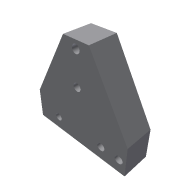
# Autodesk Inventor part: cellSTORM_chip_Adapter_screws
Saved by Autodesk Inventor 2019 (Build 230136000, 136)
## iProperties
Created: 2020-02-12
Part Number: cellSTORM_chip_Adapter_screws
Material: Generic
Document SubType Name: Modeling
Designer: diederichbenedict
Density: 1 g/cm^3
Appearance: Default
Author: diederichbenedict
Autodesk Inventor part; units mm, degrees
ref_plane "YZ Plane" through (0, 0, 0) normal (1, 0, 0) x (0, 1, 0)
ref_plane "XZ Plane" through (0, 0, 0) normal (0, 1, 0) x (-1, 0, 0)
ref_plane "XY Plane" through (0, 0, 0) normal (0, 0, 1) x (1, 0, 0)
sketch "Sketch1" plane through (0, 0, 0) normal (0, 0, 1) x (1, 0, 0)
  line L0 (18.5, -17.5) -> (-18.5, -17.5)
  line L1 (-18.5, -17.5) -> (-18.5, 17.5)
  line L2 (-18.5, 17.5) -> (18.5, 17.5)
  line L3 (18.5, 17.5) -> (18.5, -17.5)
  line L4 (18.5, -17.5) -> (-18.5, 17.5) construction
  line L5 (-18.5, -17.5) -> (18.5, 17.5) construction
  line L6 (0, 14.9312) -> (16, -12.7816) construction
  line L7 (16, -12.7816) -> (-16, -12.7816) construction
  line L8 (-16, -12.7816) -> (0, 14.9312) construction
  line L9 (-9.3116, -12.7816) -> (0.017, 3.3758) construction
  line L10 (0.017, 3.3758) -> (9.3455, -12.7816) construction
  line L11 (9.3455, -12.7816) -> (-9.3116, -12.7816) construction
  circle A0 centre (0, 14.9312) radius 1.4
  circle A1 centre (16, -12.7816) radius 1.4
  circle A2 centre (9.3455, -12.7816) radius 1.4
  circle A3 centre (0.017, 3.3758) radius 1.4
  circle A4 centre (-9.3116, -12.7816) radius 1.4
  line L12 (-4.6002, 17.5) -> (-18.5, -6.5752)
  line L13 (18.5, -6.5752) -> (4.6002, 17.5)
  point P0 (0, 0)
  point P1 (0, -3.544)
  point P2 (0.017, -7.3958)
  dimension "d0" = 37
  dimension "d1" = 35
  dimension "d3" = 32
  dimension "d4" = 0
  dimension "d5" = 2.8
  dimension "d6" = 2.8
  dimension "d7" = 2.8
  dimension "d8" = 2.8
  dimension "d9" = 2.8
  constraints: 28 end point, 5 centre point, 5 coincident, 5 parallel, 4 point on line, 2 midpoint, 1 collinear, 1 horizontal, 1 perpendicular, 14 other
  measures "d0" distance of L1.end L2.end
  measures "d1" distance of L0.end L1.end
  measures "d3" distance of L6.end L7.end
  measures "d4" distance between parallel lines of L7 L11
  measures "d5" diameter of A0
  measures "d6" diameter of A1
  measures "d7" diameter of A2
  measures "d8" diameter of A3
  measures "d9" diameter of A4
extrude "Extrusion1" add sketch "Sketch1" along normal blind 10 contours L0 L1 L12 L2 L13 L3
body "Solid1"
